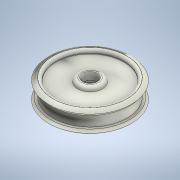
# Autodesk Inventor part: kolo_mensi
Saved by Autodesk Inventor 2022 (Build 260153000, 153)
## iProperties
Created: 2022-11-21
Part Number: kolo_mensi
Material: Generic
Document SubType Name: Modeling
Designer: matys
Density: 1 g/cm^3
Appearance: Honed
Author: matys
Autodesk Inventor part; units mm, degrees
ref_plane "YZ Plane" through (0, 0, 0) normal (1, 0, 0) x (0, 1, 0)
ref_plane "XZ Plane" through (0, 0, 0) normal (0, 1, 0) x (-1, 0, 0)
ref_plane "XY Plane" through (0, 0, 0) normal (0, 0, 1) x (1, 0, 0)
sketch "Sketch1" plane through (0, 0, 0) normal (0, 1, 0) x (-1, 0, 0)
  line L0 (0, 0) -> (17, 0)
  circle A0 centre (0, 0) radius 17
  dimension "d0" = 17
  constraints: 2 end point, 1 coincident, 1 horizontal, 1 horizontal alignment, 2 other
  measures "d0" distance of L0.start L0.end
extrude "Extrusion1" add sketch "Sketch1" along normal blind 2
sketch "Sketch2" plane through (0, 2, 0) normal (0, 1, 0) x (1, 0, 0)
  line L0 (0, 0) -> (-15, 0)
  circle A0 centre (0, 0) radius 15
  dimension "d3" = 15
  constraints: 2 end point, 1 coincident, 1 horizontal, 1 horizontal alignment, 2 other
  measures "d3" distance of L0.start L0.end
extrude "Extrusion2" add sketch "Sketch2" along normal blind 4.8
sketch "Sketch3" plane through (0, 6.8, 0) normal (0, 1, 0) x (1, 0, 0)
  circle A0 centre (0, 0) radius 17
  constraints: 1 centre point, 1 coincident
extrude "Extrusion3" add sketch "Sketch3" along normal blind 2
fillet "Fillet1" radius 2 2 edges at (-17, 8.8, 0) (17, 0, 0)
chamfer "Chamfer1" distance 1 angle 45 4 edges at (-17, 6.8001, 0) (-17, 6.8, 0) (17, 2, 0) (17, 1.9999, 0)
sketch "Sketch4" plane through (0, 8.8, 0) normal (0, 1, 0) x (1, 0, 0)
  circle A0 centre (0, 0) radius 13.75
  circle A1 centre (0, 0) radius 5
  dimension "d12" = 27.5
  dimension "d13" = 10
  constraints: 2 centre point, 2 coincident
  measures "d12" diameter of A0
  measures "d13" diameter of A1
extrude "Extrusion4" cut sketch "Sketch4" against normal blind 1.5
fillet "Fillet2" radius 1.2 1 edges at (-13.75, 8.8, 0)
fillet "Fillet3" radius 1.5 1 edges at (-5, 8.8, 0)
sketch "Sketch5" plane through (0, 8.8, 0) normal (0, 1, 0) x (1, 0, 0)
  circle A0 centre (0, 0) radius 3.5 projected
  circle A1 centre (0, 0) radius 3
  dimension "d18" = 6
  constraints: 1 centre point, 1 coincident
  measures "d18" diameter of A1
extrude "Extrusion5" cut sketch "Sketch5" against normal blind 3.2 contours A1
sketch "Sketch6" plane through (0, 5.6, 0) normal (0, 1, 0) x (1, 0, 0)
  circle A0 centre (0, 0) radius 2
  dimension "d21" = 4
  constraints: 1 centre point, 1 coincident
  measures "d21" diameter of A0
extrude "Extrusion6" cut sketch "Sketch6" against normal blind 5
sketch "Sketch7" plane through (0, 0.6, 0) normal (0, 1, 0) x (1, 0, 0)
  circle A0 centre (0, 0) radius 2 projected
  line L0 (0, -2) -> (-2, 0)
  line L1 (-2, 0) -> (0, 2)
  line L2 (0, 2) -> (2, 0)
  line L3 (2, 0) -> (0, -2)
  constraints: 8 end point, 2 parallel, 2 point on circle, 1 perpendicular
extrude "Extrusion7" cut sketch "Sketch7" against normal blind 5 contours L3 L0 L1 L2
body "Solid1"
